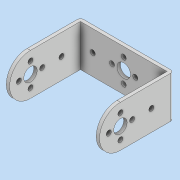
# Autodesk Inventor part: Bracket U CORTO
Saved by Autodesk Inventor 2021.4 (Build 254397000, 397)
## iProperties
Created: 2022-07-25
Part Number: Bracket U CORTO
Material: Generic
Document SubType Name: Modeling
Designer: ferbm
Density: 1 g/cm^3
Appearance: Default
Author: ferbm
Autodesk Inventor part; units mm, degrees
ref_plane "YZ Plane" through (0, 0, 0) normal (1, 0, 0) x (0, 1, 0)
ref_plane "XZ Plane" through (0, 0, 0) normal (0, 1, 0) x (-1, 0, 0)
ref_plane "XY Plane" through (0, 0, 0) normal (0, 0, 1) x (1, 0, 0)
sketch "Sketch1" plane through (0, 0, 0) normal (0, 0, 1) x (1, 0, 0)
  line L0 (0, 0) -> (52, 0)
  line L1 (52, 0) -> (52, 25)
  line L2 (52, 25) -> (0, 25)
  line L3 (0, 25) -> (0, 0)
  circle A0 centre (26, 19.5) radius 1.5
  circle A1 centre (19, 12.5) radius 1.5
  circle A2 centre (33, 12.5) radius 1.5
  circle A3 centre (26, 5.5) radius 1.5
  circle A4 centre (7.4, 12.5) radius 1.5
  circle A5 centre (44.6, 12.5) radius 1.5
  circle A6 centre (26, 12.5) radius 4.0289
  line L4 (52, 25) -> (54, 25)
  line L5 (54, 25) -> (54, 0)
  line L6 (54, 0) -> (52, 0)
  line L7 (52, 0) -> (52, 25)
  line L8 (0, 25) -> (-2, 25)
  line L9 (-2, 25) -> (-2, 0)
  line L10 (-2, 0) -> (0, 0)
  line L11 (0, 0) -> (0, 25)
  dimension "d0" = 52
  dimension "d1" = 25
  dimension "d2" = 3
  dimension "d3" = 3
  dimension "d4" = 3
  dimension "d5" = 3
  dimension "d6" = 3
  dimension "d7" = 3
  dimension "d9" = 7.4
  dimension "d10" = 7.4
  dimension "d11" = 26
  dimension "d13" = 2
  dimension "d14" = 2
  constraints: 24 end point, 7 centre point, 6 parallel, 3 horizontal, 3 perpendicular, 1 point on line
  measures "d0" distance of L1.end L2.end
  measures "d1" distance of L0.end L1.end
  measures "d2" diameter of A0
  measures "d3" diameter of A2
  measures "d4" diameter of A5
  measures "d5" diameter of A3
  measures "d6" diameter of A1
  measures "d7" diameter of A4
  measures "d9" distance from line of L1 A5.centre
  measures "d10" distance from line of L3 A4.centre
  measures "d11" distance from line of L3 A6.centre
  measures "d13" distance of L2.end L8.end
  measures "d14" distance of L1.end L4.end
extrude "Extrusion1" add sketch "Sketch1" along normal blind 2 contours L3 L2 L1 L0
extrude "Extrusion2" add sketch "Sketch1" along normal blind 3 contours L10 L9 L8 L3 | L1 L4 L5 L6
sketch "Sketch2" plane through (0, 0, 3) normal (0, 0, 1) x (1, 0, 0)
  line L0 (54, 25) -> (-2, 25) projected
  line L1 (0, 0) -> (0, 25) projected
  line L2 (-2, 25) -> (0, 25)
  line L3 (0, 25) -> (0, 0)
  line L4 (0, 0) -> (-2, 0)
  line L5 (-2, 0) -> (-2, 25)
  line L6 (52, 25) -> (52, 0) projected
  line L7 (54, 0) -> (54, 25) projected
  line L8 (52, 25) -> (54, 25)
  line L9 (54, 25) -> (54, 0)
  line L10 (54, 0) -> (52, 0)
  line L11 (52, 0) -> (52, 25)
  constraints: 16 end point, 4 parallel, 2 horizontal, 2 perpendicular
extrude "Extrusion3" add sketch "Sketch2" along normal blind 29
sketch "Sketch3" plane through (54, 0, 0) normal (1, 0, 0) x (0, 0, -1)
  line L0 (-32, 0) -> (-32, 25) projected
  line L1 (-2, 25) -> (-32, 25) projected
  line L2 (-2, 0) -> (-32, 0) projected
  arc A0 (-32, 25) -> (-32, 0) centre (-32, 12.5) ccw
  line L3 (-32, 0) -> (-32, 25) projected
  point P0 (0, 0)
  dimension "d22" = 12.5
  constraints: 2 point on circle, 1 centre point
  measures "d22" radius of A0
extrude "Extrusion4" add sketch "Sketch3" against normal blind 2
sketch "Sketch4" plane through (-2, 0, 0) normal (-1, 0, 0) x (0, 0, 1)
  arc A0 (32, 0) -> (32, 25) centre (32, 12.5) ccw projected
  line L0 (2, 25) -> (32, 25) projected
  arc A1 (32, 0) -> (32, 25) centre (32, 12.5) ccw
  line L1 (32, 25) -> (32, 0)
  point P0 (0, 0)
  constraints: 2 end point, 2 point on circle, 1 centre point, 1 concentric, 1 vertical
extrude "Extrusion5" add sketch "Sketch4" against normal blind 2
fillet "Fillet1" radius 2 2 edges at (54, 12.5, 0) (-2, 12.5, 0)
sketch "Sketch5" plane through (-2, 12.5, 32) normal (-1, 0, 0) x (0, 0, 1)
  circle A0 centre (0, 0) radius 4
  circle A1 centre (0, 0) radius 7
  circle A2 centre (0, 7) radius 1.5
  circle A3 centre (-7, 0) radius 1.5
  circle A4 centre (0, -7) radius 1.5
  circle A5 centre (7, 0) radius 1.5
  circle A6 centre (-18.6, 0) radius 1.3978
  point P0 (-32, -12.5)
  dimension "d29" = 14
  dimension "d28" = 8
  dimension "d32" = 360
  dimension "d34" = 3
  dimension "d35" = 18.6
  constraints: 6 centre point, 1 coincident, 1 vertical alignment, 11 other
  measures "d28" diameter of A0
  measures "d34" diameter of A2
  measures "d35" distance of A6.centre A0.centre
hole "Hole1" at (-2, 12.5, 32) at (-2, 12.5, 25) at (-2, 19.5, 32) at (-2, 12.5, 39) at (-2, 5.5, 32) at (-2, 12.5, 13.4) direction (1, 0, 0) diameter 3 end through all
hole "Hole2" at (-2, 12.5, 32) direction (1, 0, 0) diameter 8 end through all
body "Solid1"
